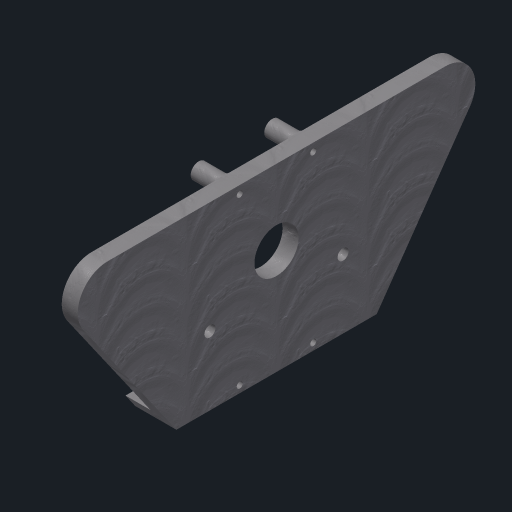
# Autodesk Inventor part: CAJA
Saved by Autodesk Inventor 2024.3 (Build 283343000, 343)
## iProperties
Created: 2024-06-29
Part Number: CAJA
Material: Steel, Mild, Welded
Document SubType Name: Modeling
Designer: Niler
Density: 7.85 g/cm^3
Appearance: Weld - Steel Mild
Author: Niler
Autodesk Inventor part; units mm, degrees
ref_plane "YZ Plane" through (0, 0, 0) normal (1, 0, 0) x (0, 1, 0)
ref_plane "XZ Plane" through (0, 0, 0) normal (0, 1, 0) x (-1, 0, 0)
ref_plane "XY Plane" through (0, 0, 0) normal (0, 0, 1) x (1, 0, 0)
sketch "Sketch1" plane through (0, 0, 0) normal (1, 0, 0) x (0, 1, 0)
  line L0 (-67.5, 145) -> (67.5, 145)
  line L1 (67.5, 145) -> (67.5, -145)
  line L2 (67.5, -145) -> (-67.5, -145)
  line L3 (-67.5, -145) -> (-67.5, 145)
  line L4 (-67.5, 145) -> (67.5, -145) construction
  line L5 (67.5, 145) -> (-67.5, -145) construction
  circle A0 centre (0, 77.5) radius 3.925
  circle A1 centre (0, -77.5) radius 3.925
  circle A2 centre (-15, 0) radius 5
  line L6 (0, 77.5) -> (0, -77.5) construction
  line L7 (60.5, -138) -> (60.5, 138)
  line L8 (60.5, 138) -> (-60.5, 138)
  line L9 (-60.5, 138) -> (-60.5, -138)
  line L10 (-60.5, -138) -> (60.5, -138)
  point P0 (0, 0)
  dimension "d0" = 155
  dimension "d1" = 7.85
  dimension "d2" = 290
  dimension "d3" = 135
  dimension "d4" = 7
  dimension "d35" = 10
  dimension "d36" = 15
  constraints: 22 end point, 4 parallel, 3 centre point, 3 midpoint, 2 perpendicular, 1 equal radius, 1 horizontal, 1 horizontal alignment, 1 vertical, 1 vertical alignment, 3 other
  measures "d0" distance of L6.end L6.start
  measures "d1" diameter of A0
  measures "d2" distance between parallel lines of L2 L0
  measures "d3" distance of L0.start L0.end
  measures "d4" distance between parallel lines of L1 L7
  measures "d35" diameter of A2
  measures "d36" distance of A2.centre point (0, 0)
extrude "Extrusion1" add sketch "Sketch1" along normal blind 8 contours L0 L1 L2 L3 | A0 | A1 | L10 L9 L8 L7
extrude "Extrusion2" add sketch "Sketch1" against normal blind 12.5 contours L0 L1 L2 L3 | A0 | A1
sketch "Sketch2" plane through (8, 0, 0) normal (1, 0, 0) x (0, 0, -1)
  line L0 (145, -67.5) -> (145, 67.5) projected
  line L1 (145, 67.5) -> (-145, 67.5) projected
  line L2 (-145, 67.5) -> (-145, -67.5) projected
  line L3 (-145, -67.5) -> (145, -67.5) projected
  line L4 (-33.234, -33.234) -> (33.234, -33.234) construction
  line L5 (33.234, -33.234) -> (33.234, 33.234) construction
  line L6 (33.234, 33.234) -> (-33.234, 33.234) construction
  line L7 (-33.234, 33.234) -> (-33.234, -33.234) construction
  line L8 (-33.234, -33.234) -> (33.234, 33.234) construction
  line L9 (33.234, -33.234) -> (-33.234, 33.234) construction
  circle A0 centre (0, 0) radius 47 construction
  circle A1 centre (33.234, 33.234) radius 2.75
  circle A2 centre (-33.234, 33.234) radius 2.75
  circle A3 centre (0, 0) radius 47 construction
  circle A4 centre (-33.234, -33.234) radius 2.75
  circle A5 centre (0, 0) radius 47 construction
  circle A6 centre (33.234, -33.234) radius 2.75
  circle A7 centre (0, 0) radius 47 construction
  point P0 (0, 0)
  point P1 (0, 0)
  dimension "d12" = 94
  dimension "d13" = 5.5
  dimension "d16" = 360
  constraints: 12 end point, 7 coincident, 4 centre point, 2 parallel, 2 perpendicular, 1 horizontal, 1 midpoint, 31 other
  measures "d13" diameter of A1
extrude "Extrusion3" cut sketch "Sketch2" against normal through all contours A1 | A2 | A4 | A6
sketch "Sketch3" plane through (0, 0, 0) normal (-1, 0, 0) x (0, 0, 1)
  circle A0 centre (33.234, -33.234) radius 2.75 projected
  circle A1 centre (33.234, 33.234) radius 2.75 projected
  circle A2 centre (-33.234, -33.234) radius 2.75 projected
  circle A3 centre (-33.234, 33.234) radius 2.75 projected
  line L0 (-138, -60.5) -> (138, -60.5) projected
  line L1 (138, -60.5) -> (138, 60.5) projected
  line L2 (138, 60.5) -> (-138, 60.5) projected
  line L3 (-138, 60.5) -> (-138, -60.5) projected
  circle A4 centre (77.5, 0) radius 3.925 projected
  circle A5 centre (-77.5, 0) radius 3.925 projected
  circle A6 centre (0, -15) radius 5 projected
  circle A7 centre (-33.234, 33.234) radius 4.5
  circle A8 centre (33.234, 33.234) radius 2.75 projected
  circle A9 centre (33.234, 33.234) radius 4.5
  circle A10 centre (-33.234, -33.234) radius 4.5
  circle A11 centre (33.234, -33.234) radius 4.5
  point P0 (0, 0)
  dimension "d20" = 9
  constraints: 4 centre point, 4 coincident, 3 equal radius
  measures "d20" diameter of A7
extrude "Extrusion4" cut sketch "Sketch3" against normal blind 3 contours A0 | A1 | A2 | A3 | A7 | A9 | A10 | A11
fillet "Fillet1" radius 2 2 edges at (0, -3.925, -77.5) (0, -3.925, 77.5)
sketch "Sketch4" plane through (8, 0, 0) normal (1, 0, 0) x (0, 0, -1)
  circle A0 centre (-33.234, -33.234) radius 2.75 projected
  circle A1 centre (-33.234, 33.234) radius 2.75 projected
  circle A2 centre (33.234, -33.234) radius 2.75 projected
  circle A3 centre (33.234, 33.234) radius 2.75 projected
  line L0 (145, -67.5) -> (145, 67.5) projected
  line L1 (145, 67.5) -> (-145, 67.5) projected
  line L2 (-145, 67.5) -> (-145, -67.5) projected
  line L3 (-145, -67.5) -> (145, -67.5) projected
  circle A4 centre (0, -15) radius 5 projected
  circle A5 centre (0, -15) radius 11
  point P0 (0, 0)
  dimension "d24" = 22
  constraints: 1 centre point, 1 coincident
  measures "d24" diameter of A5
extrude "Extrusion5" cut sketch "Sketch4" against normal through all contours A4 | A5
sketch "Sketch5" plane through (-12.5, 0, -77.5) normal (-1, 0, 0) x (0, 0, 1)
  circle A0 centre (0, 0) radius 3.925 projected
  circle A1 centre (155, 0) radius 3.925 projected
  point P0 (77.5, 0)
extrude "Extrusion6" cut sketch "Sketch5" against normal blind 2.5
chamfer "Chamfer2" distance 20 angle 45 8 edges at (-6.25, 60.5, -138) (-6.25, -60.5, -138) (-6.25, -60.5, 138) (-6.25, 60.5, 138) (-2.25, 67.5, -145) (-2.25, -67.5, -145) (-2.25, -67.5, 145) (-2.25, 67.5, 145)
sketch "Sketch6" plane through (-12.5, 0, 0) normal (-1, 0, 0) x (0, 0, 1)
  line L0 (125, 67.5) -> (145, 47.5) projected
  line L1 (125, 67.5) -> (-125, 67.5) projected
  line L2 (-145, 47.5) -> (-125, 67.5) projected
  line L3 (-145, 47.5) -> (-145, -47.5) projected
  line L4 (-125, -67.5) -> (-145, -47.5) projected
  line L5 (-125, -67.5) -> (125, -67.5) projected
  line L6 (145, -47.5) -> (125, -67.5) projected
  line L7 (145, -47.5) -> (145, 47.5) projected
  line L8 (-138, -40.5) -> (-138, 40.5) projected
  line L9 (-118, 60.5) -> (-138, 40.5) projected
  line L10 (-118, 60.5) -> (118, 60.5) projected
  line L11 (138, 40.5) -> (118, 60.5) projected
  line L12 (138, 40.5) -> (138, -40.5) projected
  line L13 (118, -60.5) -> (138, -40.5) projected
  line L14 (118, -60.5) -> (-118, -60.5) projected
  line L15 (-138, -40.5) -> (-118, -60.5) projected
  line L16 (131.5, -54) -> (-131.5, -54)
  line L17 (-131.5, -54) -> (-131.5, 54)
  line L18 (-131.5, 54) -> (131.5, 54)
  line L19 (131.5, 54) -> (131.5, -54)
  circle A0 centre (0, 0) radius 10.3
  line L20 (131.5, -54) -> (-131.5, 54) construction
  line L21 (-131.5, -54) -> (131.5, 54) construction
  circle A1 centre (-131.5, 54) radius 1.5
  circle A2 centre (-131.5, -54) radius 1.5
  circle A3 centre (131.5, -54) radius 1.5
  circle A4 centre (131.5, 54) radius 1.5
  line L22 (-135, 57.5) -> (-128, 50.5)
  dimension "d32" = 3
  constraints: 14 end point, 5 centre point, 5 coincident, 5 midpoint, 3 equal radius, 2 parallel, 1 horizontal, 1 perpendicular
  measures "d32" diameter of A1
extrude "Extrusion7" cut sketch "Sketch6" against normal through all contours A2 L16 L17 | L17 L16 A2 | A1 L22 L17 | L17 L22 A1 | L22 L18 A1 | L22 A1 L18 | A3 L19 L16 | L16 L19 A3 | A4 L19 L18 | L18 L19 A4
sketch "Sketch7" plane through (8, 0, 0) normal (1, 0, 0) x (0, 0, -1)
  circle A0 centre (-131.5, -54) radius 1.5 projected
  circle A1 centre (131.5, -54) radius 1.5 projected
  circle A2 centre (-131.5, 54) radius 1.5 projected
  circle A3 centre (131.5, 54) radius 1.5 projected
  line L0 (-145, 47.5) -> (-125, 67.5) projected
  line L1 (-145, 47.5) -> (-145, -47.5) projected
  line L2 (-125, -67.5) -> (-145, -47.5) projected
  line L3 (-125, -67.5) -> (125, -67.5) projected
  line L4 (145, -47.5) -> (125, -67.5) projected
  line L5 (145, -47.5) -> (145, 47.5) projected
  line L6 (125, 67.5) -> (145, 47.5) projected
  line L7 (125, 67.5) -> (-125, 67.5) projected
  circle A4 centre (0, -15) radius 11 projected
  circle A5 centre (-33.234, -33.234) radius 2.75 projected
  circle A6 centre (-33.234, 33.234) radius 2.75 projected
  circle A7 centre (33.234, -33.234) radius 2.75 projected
  circle A8 centre (33.234, 33.234) radius 2.75 projected
  circle A9 centre (-77.5, 0) radius 3.925 projected
  circle A10 centre (-77.5, 0) radius 3.925 projected
  circle A11 centre (77.5, 0) radius 3.925 projected
  circle A12 centre (77.5, 0) radius 3.925 projected
  line L8 (-50, -67.5) -> (-96.4912, -1.1036)
  line L9 (-84.2039, 22.5) -> (0, 22.5)
  line L10 (0, 22.5) -> (0, -67.5)
  arc A13 (-84.2039, 22.5) -> (-96.4912, -1.1036) centre (-84.2039, 7.5) ccw
  line L11 (-125, -67.5) -> (125, -67.5) projected
  line L12 (50, -67.5) -> (96.4912, -1.1036)
  line L13 (84.2039, 22.5) -> (0, 22.5)
  arc A14 (96.4912, -1.1036) -> (84.2039, 22.5) centre (84.2039, 7.5) ccw
  point P0 (0, 0)
  point P1 (0, -67.5)
  point P2 (0, -67.5)
  point P3 (50, -67.5)
  dimension "d37" = 15
  dimension "d38" = 90
  dimension "d39" = 50
  dimension "d40" = 55
  constraints: 10 end point, 4 point on circle, 4 symmetric about line, 3 midpoint, 2 centre point, 2 tangent, 1 horizontal, 1 point on line, 1 vertical alignment, 1 other
  measures "d37" radius of A13
  measures "d38" distance of L9.end L10.end
  measures "d39" distance of point (0, -67.5) L8.start
  measures "d40" angle of L3 L8
extrude "Extrusion8" cut sketch "Sketch7" against normal through all contours L0 L7 L6 L5 L4 L3 L12 A14 L13 L9 A13 L8 L2 L1
sketch "Sketch8" plane through (0, 0, 0) normal (-1, 0, 0) x (0, 0, 1)
  circle A0 centre (-77.5, 0) radius 3.925 projected
  circle A1 centre (77.5, 0) radius 3.925 projected
  circle A2 centre (-77.5, 0) radius 53
  line L0 (54.9015, -60.5) -> (96.4912, -1.1036) projected
  arc A3 (96.4912, -1.1036) -> (84.2039, 22.5) centre (84.2039, 7.5) ccw projected
  line L1 (84.2039, 22.5) -> (-84.2039, 22.5) projected
  arc A4 (-84.2039, 22.5) -> (-96.4912, -1.1036) centre (-84.2039, 7.5) ccw projected
  line L2 (-96.4912, -1.1036) -> (-54.9015, -60.5) projected
  line L3 (-54.9015, -60.5) -> (54.9015, -60.5) projected
  circle A5 centre (0, -15) radius 11 projected
  circle A6 centre (-77.5, 0) radius 5.925 projected
  circle A7 centre (-33.234, -33.234) radius 4.5 projected
  circle A8 centre (33.234, -33.234) radius 4.5 projected
  circle A9 centre (77.5, 0) radius 5.925 projected
  circle A10 centre (-18.3535, 18.5) radius 4
  line L4 (84.2039, 22.5) -> (-84.2039, 22.5) projected
  line L5 (0, 0) -> (0, 7.5)
  circle A11 centre (18.3535, 18.5) radius 4
  circle A12 centre (0, -15) radius 25.9383
  dimension "d43" = 106
  dimension "d44" = 8
  constraints: 4 centre point, 3 coincident, 2 end point, 2 tangent, 1 symmetric about line, 1 vertical, 1 other
  measures "d43" diameter of A2
  measures "d44" diameter of A10
extrude "Extrusion9" add sketch "Sketch8" along normal up to surface (12.5 mm away) contours A11 | A10
fillet "Fillet2" radius 2 4 edges at (0, 21.3284, -15.5251) (0, 15.6716, -21.1819) (0, 21.3284, 21.1819) (0, 15.6716, 15.5251)
sketch "Sketch9" plane through (-12.5, 18.5, 18.3535) normal (-1, 0, 0) x (0, 0, 1)
  circle A0 centre (-36.707, 0) radius 4 projected
  circle A1 centre (0, 0) radius 4 projected
  circle A2 centre (-36.707, 0) radius 1.5
  circle A3 centre (0, 0) radius 1.5
  line L0 (31.6465, -86) -> (36.5479, -79) projected
  line L1 (36.5479, -79) -> (-73.255, -79) projected
  line L2 (-73.255, -79) -> (-68.3535, -86) projected
  line L3 (-68.3535, -86) -> (31.6465, -86) projected
  circle A4 centre (-36.707, -82.5) radius 1.5
  circle A5 centre (0, -82.5) radius 1.5
  point P0 (-18.3535, -18.5)
  point P1 (-70.8042, -82.5)
  dimension "d48" = 3
  dimension "d49" = 3
  dimension "d52" = 3
  dimension "d53" = 3
  constraints: 4 centre point, 2 coincident, 2 horizontal alignment, 2 vertical alignment, 1 midpoint
  measures "d48" diameter of A2
  measures "d49" diameter of A3
  measures "d52" diameter of A4
  measures "d53" diameter of A5
extrude "Extrusion10" cut sketch "Sketch9" against normal through all contours A2 | A3 | A4 | A5
body "Solid1"
